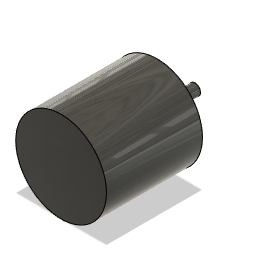
9V Motor_ (Autodesk Fusion 360 design; units mm, degrees)
Autodesk Fusion 360 part; units mm, degrees
sketch "Sketch1" plane through (0, 0, 0) normal (0, 0, 1) x (1, 0, 0)
  circle A0 centre (220, 20) radius 12
  dimension "d31_1" = 24
  measures "d31_1" diameter of A0
extrude "Extrude1" add sketch "Sketch1" along normal blind 25.4
sketch "Sketch2" plane through (0, 0, 0) normal (0, 0, -1) x (-1, 0, 0)
  circle A0 centre (-220, 20) radius 12
  circle A1 centre (-220, 20) radius 1.5
  dimension "d34_1" = 3
  constraint concentric A0 A1
  measures "d34_1" diameter of A1
extrude "Extrude2" add sketch "Sketch2" along normal blind 10 contours A1
